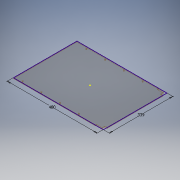
# Autodesk Inventor part: Acrylic_Panel
Saved by Autodesk Inventor 2019.4 (Build 234330000, 330)
## iProperties
Created: 2020-01-31
Part Number: Acrylic_Panel
Material: Generic
Document SubType Name: Modeling
Designer: Jorian Bruslind
Density: 1 g/cm^3
Appearance: Polycarbonate - Smoked
Author: Jorian Bruslind
Autodesk Inventor part; units mm, degrees
ref_plane "YZ Plane" through (0, 0, 0) normal (1, 0, 0) x (0, 1, 0)
ref_plane "XZ Plane" through (0, 0, 0) normal (0, 1, 0) x (-1, 0, 0)
ref_plane "XY Plane" through (0, 0, 0) normal (0, 0, 1) x (1, 0, 0)
sketch "Sketch1" plane through (0, 0, 0) normal (0, 1, 0) x (-1, 0, 0)
  line L0 (-240, 168.915) -> (240, 168.915)
  line L1 (240, 168.915) -> (240, -168.915)
  line L2 (240, -168.915) -> (-240, -168.915)
  line L3 (-240, -168.915) -> (-240, 168.915)
  line L4 (-240, 168.915) -> (240, -168.915) construction
  line L5 (240, 168.915) -> (-240, -168.915) construction
  point P0 (0, 0)
  dimension "d0" = 480
  dimension "d1" = 337.83
  constraints: 12 end point, 2 midpoint, 2 parallel, 1 horizontal, 1 perpendicular
  measures "d0" distance of L1.end L2.end
  measures "d1" distance of L0.end L1.end
extrude "Extrusion1" add sketch "Sketch1" along normal blind 5
sketch "Sketch2" plane through (0, 5, 0) normal (0, 1, 0) x (1, 0, 0)
  line L0 (240, -168.915) -> (240, 168.915) projected
  line L1 (240, -168.915) -> (240, -148.915)
  line L2 (240, -148.915) -> (228, -148.915)
  line L3 (-240, -168.915) -> (240, -168.915) projected
  line L4 (228, -168.915) -> (228, -163.915)
  line L5 (228, -168.915) -> (233, -168.915) construction
  line L6 (228, -148.915) -> (228, -163.915)
  line L7 (228, -163.915) -> (196, -163.915)
  line L8 (196, -163.915) -> (196, -168.915)
  line L9 (196, -168.915) -> (240, -168.915)
  line L10 (240, 0) -> (160.3142, 0)
  line L11 (240, 168.915) -> (240, 148.915)
  line L12 (240, 148.915) -> (228, 148.915)
  line L13 (228, 168.915) -> (228, 163.915)
  line L14 (228, 168.915) -> (233, 168.915) construction
  line L15 (228, 148.915) -> (228, 163.915)
  line L16 (228, 163.915) -> (196, 163.915)
  line L17 (196, 163.915) -> (196, 168.915)
  line L18 (196, 168.915) -> (240, 168.915)
  point P0 (0, 0)
  dimension "d4" = 20
  dimension "d5" = 12
  dimension "d6" = 5
  dimension "d7" = 90
  dimension "d8" = 15
  dimension "d9" = 32
  constraints: 34 end point, 7 symmetric about line, 5 perpendicular, 3 horizontal, 3 point on line, 1 midpoint, 1 vertical
  measures "d4" distance of L0.start L1.end
  measures "d5" distance of L1.end L2.end
  measures "d6" distance of L4.start L4.end
  measures "d7" angle of L5 L4
  measures "d8" distance of L2.end L4.end
  measures "d9" distance of L4.end L7.end
extrude "Extrusion2" cut sketch "Sketch2" against normal blind 5
sketch "Sketch4" plane through (0, 5, 0) normal (0, 1, 0) x (1, 0, 0)
  line L0 (-240, -168.915) -> (196, -168.915) projected
  line L1 (-240, -168.915) -> (-200, -168.915)
  line L2 (-200, -168.915) -> (-200, -160.183)
  circle A0 centre (-200, -160.183) radius 2.75
  circle A1 centre (-100, -160.183) radius 2.75
  circle A2 centre (0, -160.183) radius 2.75
  circle A3 centre (100, -160.183) radius 2.75
  line L3 (196, 168.915) -> (-240, 168.915) projected
  line L4 (-240, 168.915) -> (-180, 168.915)
  line L5 (-180, 168.915) -> (-180, 160.183)
  circle A4 centre (-180, 160.183) radius 2.75
  circle A5 centre (-80, 160.183) radius 2.75
  circle A6 centre (20, 160.183) radius 2.75
  circle A7 centre (120, 160.183) radius 2.75
  point P0 (0, 0)
  dimension "d14" = 40
  dimension "d15" = 8.732
  dimension "d16" = 5.5
  dimension "d19" = 100
  dimension "d24" = 60
  dimension "d25" = 8.732
  dimension "d26" = 5.5
  dimension "d29" = 100
  constraints: 8 centre point, 8 end point, 2 coincident, 2 horizontal, 2 perpendicular, 2 point on line, 12 other
  measures "d14" distance of L0.start L1.end
  measures "d15" distance of L1.end L2.end
  measures "d16" diameter of A0
  measures "d19" distance of A0.centre A1.centre
  measures "d24" distance of L3.end L4.end
  measures "d25" distance of L4.end L5.end
  measures "d26" diameter of A4
  measures "d29" distance of A4.centre A5.centre
extrude "Extrusion3" cut sketch "Sketch4" against normal blind 10
sketch "Sketch5" plane through (0, 5, 0) normal (0, 1, 0) x (1, 0, 0)
  line L0 (196, 168.915) -> (-240, 168.915) projected
  line L1 (-240, 168.915) -> (240, 168.915)
  line L2 (240, 168.915) -> (240, -170.085)
  line L3 (240, -170.085) -> (-240, -170.085)
  line L4 (-240, -170.085) -> (-240, 168.915)
  point P0 (0, 0)
  dimension "d36" = 480
  dimension "d37" = 339
  constraints: 8 end point, 2 parallel, 1 horizontal, 1 perpendicular
  measures "d36" distance of L2.end L3.end
  measures "d37" distance of L1.end L2.end
body "Solid1"
